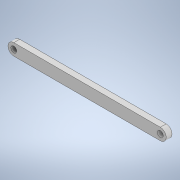
# Autodesk Inventor part: Biela
Saved by Autodesk Inventor 2020 (Build 240168000, 168)
## iProperties
Created: 2020-11-30
Part Number: Biela
Material: Generic
Document SubType Name: Modeling
Designer: Daniel
Density: 1 g/cm^3
Appearance: Default
Author: Daniel
Autodesk Inventor part; units mm, degrees
ref_plane "YZ Plane" through (0, 0, 0) normal (1, 0, 0) x (0, 1, 0)
ref_plane "XZ Plane" through (0, 0, 0) normal (0, 1, 0) x (-1, 0, 0)
ref_plane "XY Plane" through (0, 0, 0) normal (0, 0, 1) x (1, 0, 0)
sketch "Sketch1" plane through (0, 0, 0) normal (0, 0, 1) x (1, 0, 0)
  line L0 (0, 0) -> (635, 0)
  line L1 (635, 50.8) -> (0, 50.8)
  arc A0 (635, 0) -> (635, 50.8) centre (635, 25.4) ccw
  arc A1 (0, 50.8) -> (0, 0) centre (0, 25.4) ccw
  circle A2 centre (0, 25.4) radius 12.7
  circle A3 centre (635, 25.4) radius 12.7
  dimension "d0" = 635
  dimension "d1" = 635
  dimension "d2" = 50.8
  dimension "d3" = 25.4
  dimension "d4" = 25.4
  constraints: 4 centre point, 4 end point, 4 point on circle, 3 tangent, 2 coincident, 2 horizontal
  measures "d0" distance of L0.start L0.end
  measures "d1" distance of L1.start L1.end
  measures "d2" distance between parallel lines of L0 L1
  measures "d3" diameter of A2
  measures "d4" diameter of A3
extrude "Extrusion1" add sketch "Sketch1" along normal blind 25.4
body "Solid1"
